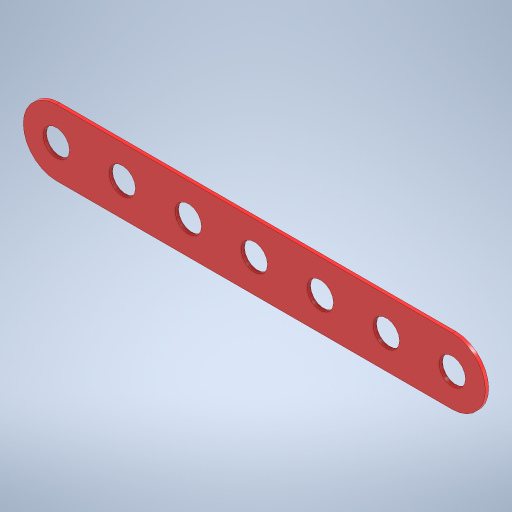
# Autodesk Inventor part: 1007
Saved by Autodesk Inventor 2024 (Build 280153000, 153)
## iProperties
Created: 2024-09-14
Part Number: 1007
Material: Všeobecné
Document SubType Name: Modeling
Designer: Student
Density: 1 g/cm^3
Appearance: Světle červená
Author: Student
Autodesk Inventor part; units mm, degrees
ref_plane "YZ Plane" through (0, 0, 0) normal (1, 0, 0) x (0, 1, 0)
ref_plane "XZ Plane" through (0, 0, 0) normal (0, 1, 0) x (-1, 0, 0)
ref_plane "XY Plane" through (0, 0, 0) normal (0, 0, 1) x (1, 0, 0)
sketch "Náčrt1" plane through (0, 0, 0) normal (0, 0, 1) x (1, 0, 0)
  line L0 (-30, 0) -> (30, 0) construction
  line L1 (-30, -5) -> (30, -5)
  line L2 (30, 5) -> (-30, 5)
  arc A0 (-30, 5) -> (-30, -5) centre (-30, 0) ccw
  arc A1 (30, -5) -> (30, 5) centre (30, 0) ccw
  point P0 (0, 0)
  point P1 (35, 0)
  dimension "d0" = 35
  dimension "d1" = 5
  constraints: 8 end point, 5 point on circle, 4 tangent, 2 centre point, 1 horizontal, 1 midpoint, 1 parallel
  measures "d0" distance of point (35, 0) point (0, 0)
  measures "d1" distance from line of L2 point (0, 0)
extrude "Vysunutí1" add sketch "Náčrt1" along normal blind 0.5
sketch "Náčrt2" plane through (0, 0, 0) normal (0, 0, -1) x (-1, 0, 0)
  arc A0 (30, -5) -> (30, 5) centre (30, 0) ccw projected
  circle A1 centre (30, 0) radius 2
  point P0 (0, 0)
  dimension "d4" = 4
  constraints: 1 centre point, 1 coincident
  measures "d4" diameter of A1
extrude "Vysunutí2" cut sketch "Náčrt2" against normal through all
pattern_linear "Obdélníkové pole1" count 7 spacing 10 along (1, 0, 0) of "Vysunutí2"
